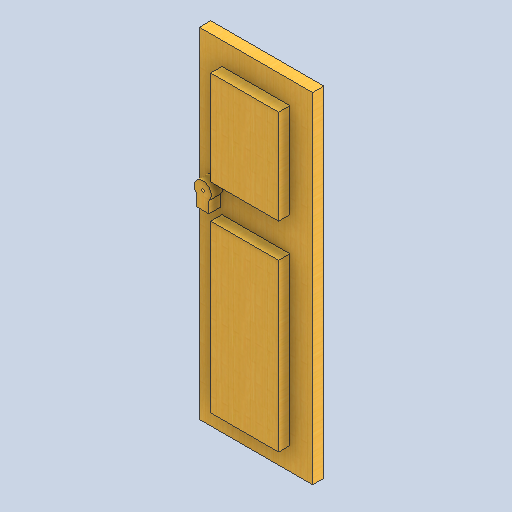
# Autodesk Inventor part: Maitri_door
Saved by Autodesk Inventor 2024.1 (Build 281209000, 209)
## iProperties
Created: 2023-10-24
Part Number: Maitri_door
Material: Bamboo
Document SubType Name: Modeling
Designer: maitr
Density: 0.7 g/cm^3
Appearance: Bamboo
Author: maitr
Autodesk Inventor part; units mm, degrees
ref_plane "YZ Plane" through (0, 0, 0) normal (1, 0, 0) x (0, 1, 0)
sketch "Sketch1" plane through (0, 0, 0) normal (0, 0, 1) x (1, 0, 0)
  line L0 (0, 0) -> (1000, 0)
  line L1 (1000, 0) -> (1000, 3000)
  line L2 (1000, 3000) -> (0, 3000)
  line L3 (0, 3000) -> (0, 0)
  dimension "d0" = 1000
  dimension "d1" = 3000
  constraints: 8 end point, 2 parallel, 1 horizontal, 1 perpendicular
  measures "d0" distance of L2.end L1.end
  measures "d1" distance of L1.end L0.end
extrude "Extrusion1" add sketch "Sketch1" along normal blind 100
ref_plane "Work Plane1" through (0, 0, 100) normal (0, 0, 1) x (1, 0, 0)
sketch "Sketch2" plane through (0, 0, 100) normal (0, 0, 1) x (1, 0, 0)
  line L0 (200, 2800) -> (800, 2800)
  line L1 (800, 2800) -> (800, 1966.6251)
  line L2 (800, 1966.6251) -> (200, 1966.6251)
  line L3 (200, 1966.6251) -> (200, 2800)
  line L4 (200, 1666.6251) -> (800, 1666.6251)
  line L5 (800, 1666.6251) -> (800, 200)
  line L6 (800, 200) -> (200, 200)
  line L7 (200, 200) -> (200, 1666.6251)
  line L8 (1000, 3000) -> (0, 3000) projected
  line L9 (0, 3000) -> (0, 0) projected
  line L10 (1000, 0) -> (1000, 3000) projected
  line L11 (0, 0) -> (1000, 0) projected
  dimension "d5" = 200
  dimension "d6" = 200
  dimension "d7" = 200
  dimension "d8" = 300
  dimension "d9" = 200
  constraints: 16 end point, 4 parallel, 2 horizontal, 2 perpendicular, 2 point on line
  measures "d5" distance between parallel lines of L0 L8
  measures "d6" distance between parallel lines of L9 L3
  measures "d7" distance between parallel lines of L10 L1
  measures "d8" distance between parallel lines of L4 L2
  measures "d9" distance between parallel lines of L11 L6
extrude "Extrusion2" add sketch "Sketch2" along normal blind 100 contours L0 L1 L2 L3 | L4 L5 L6 L7
ref_plane "Work Plane2" through (0, 0, 100) normal (0, 0, 1) x (1, 0, 0)
sketch "Sketch3" plane through (0, 0, 100) normal (0, 0, 1) x (1, 0, 0)
  circle A0 centre (130, 1866.6251) radius 75
  line L0 (200, 2800) -> (200, 1966.6251) projected
  line L1 (200, 1966.6251) -> (800, 1966.6251) projected
  line L2 (75.9991, 1814.578) -> (75.9991, 1714.578)
  line L3 (184.0009, 1814.578) -> (184.0009, 1714.578)
  line L4 (184.0009, 1714.578) -> (75.9991, 1714.578)
  point P0 (0, 0)
  dimension "d13" = 150
  dimension "d14" = 70
  dimension "d15" = 100
  dimension "d16" = 100
  dimension "d17" = 100
  constraints: 6 end point, 2 point on circle, 2 vertical, 1 centre point, 1 perpendicular
  measures "d13" diameter of A0
  measures "d14" distance from line of L0 A0.centre
  measures "d15" distance from line of A0.centre L1
  measures "d16" distance of L2.start L2.end
  measures "d17" distance of L3.start L3.end
extrude "Extrusion3" add sketch "Sketch3" along normal blind 100
sketch "Sketch4" plane through (0, 0, 200) normal (0, 0, 1) x (1, 0, 0)
  arc A0 (184.0009, 1814.578) -> (75.9991, 1814.578) centre (130, 1866.6251) ccw projected
  point P0 (0, 0)
  constraints: 1 coincident
hole "Hole1" at (130, 1866.6251, 200) direction (0, 0, -1) diameter 25 depth 100
body "Solid1"
